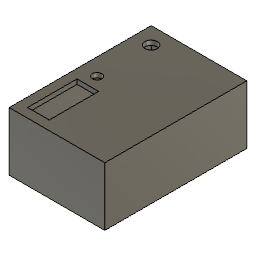
LocalMindCAD (Autodesk Fusion 360 design; units mm, degrees)
part number: 2026-03-10-18-57-42-287
Autodesk Fusion 360 part; units mm, degrees
sketch "Sketch1" plane through (0, 0, 0) normal (0, 0, 1) x (1, 0, 0)
  line L0 (31, 46) -> (-31, 46)
  line L1 (-31, 46) -> (-31, -46)
  line L2 (-31, -46) -> (31, -46)
  line L3 (31, -46) -> (31, 46)
  line L4 (31, 46) -> (-31, -46) construction
  line L5 (-31, 46) -> (31, -46) construction
  dimension "d1" = 62
  dimension "d2" = 92
  constraint horizontal L0
  constraint perpendicular L0 L1
  constraint parallel L0 L2
  constraint parallel L1 L3
  constraint coincident L4 origin
  constraint coincident L5 origin
  measures "d1" distance of L1.end L2.end
  measures "d2" distance of L0.end L1.end
extrude "Extrude1" add sketch "Sketch1" along normal blind 35
sketch "Sketch2" plane through (0, 0, 35) normal (0, 0, 1) x (-1, 0, 0)
  line L0 (-31, 46) -> (-31, -46)
  line L1 (-31, -46) -> (31, -46)
  line L2 (31, -46) -> (31, 46)
  line L3 (31, 46) -> (-31, 46)
  line L4 (31, 46) -> (-31, 46)
  line L5 (-31, 46) -> (-31, -46)
  line L6 (-31, -46) -> (31, -46)
  line L7 (31, -46) -> (31, 46)
  line L8 (29, -44) -> (29, 44)
  line L9 (29, 44) -> (-29, 44)
  line L10 (-29, 44) -> (-29, -44)
  line L11 (-29, -44) -> (29, -44)
  dimension "d5" = -2
  constraint horizontal L4
  constraint vertical L5
  constraint horizontal L6
  constraint vertical L7
  constraint coincident L0.end L1.start
  constraint coincident L2.end L3.start
extrude "Extrude2" cut sketch "Sketch2" against normal blind 33 contours L8 L9 L10 L11
sketch "Sketch3" plane through (0, 0, 2) normal (0, 0, 1) x (-1, 0, 0)
  line L0 (-29, -44) -> (29, -44)
  line L1 (29, -44) -> (29, 44)
  line L2 (29, 44) -> (-29, 44)
  line L3 (-29, 44) -> (-29, -44)
  line L4 (31, 46, 33) -> (-31, 46, 33)
  line L5 (-31, 46, 33) -> (-31, -46, 33)
  line L6 (-31, -46, 33) -> (31, -46, 33)
  line L7 (31, -46, 33) -> (31, 46, 33)
extrude "Extrude3" add sketch "Sketch3" along normal blind 3 contours L4 L5 L6 L7 in plane through (0, 0, 35) normal (0, 0, 1)
sketch "Sketch4" plane through (0, 0, 38) normal (0, 0, 1) x (-1, 0, 0)
  line L0 (31, -46) -> (31, 46)
  line L1 (31, 46) -> (-31, 46)
  line L2 (-31, 46) -> (-31, -46)
  line L3 (-31, -46) -> (31, -46)
  line L4 (25, 40) -> (11, 40)
  line L5 (11, 40) -> (11, 8)
  line L6 (11, 8) -> (25, 8)
  line L7 (25, 8) -> (25, 40)
  dimension "d10" = 14
  dimension "d11" = 32
  constraint horizontal L4
  constraint vertical L5
  constraint horizontal L6
  constraint vertical L7
  measures "d10" distance of L4.start L4.end
  measures "d11" distance of L4.start L6.end
extrude "Extrude4" cut sketch "Sketch4" against normal blind 3 contours L4 L5 L6 L7
sketch "Sketch5" plane through (0, 0, 38) normal (0, 0, 1) x (-1, 0, 0)
  line L0 (11, 40) -> (25, 40)
  line L1 (25, 40) -> (25, 8)
  line L2 (25, 8) -> (11, 8)
  line L3 (11, 8) -> (11, 40)
  line L4 (31, -46) -> (31, 46)
  line L5 (31, 46) -> (-31, 46)
  line L6 (-31, 46) -> (-31, -46)
  line L7 (-31, -46) -> (31, -46)
  circle A0 centre (20, 0) radius 3
  dimension "d14" = 6
  measures "d14" diameter of A0
extrude "Extrude5" cut sketch "Sketch5" against normal blind 3 contours A0
sketch "Sketch6" plane through (0, 0, 38) normal (0, 0, 1) x (-1, 0, 0)
  circle A0 centre (20, 0) radius 3
  line L0 (11, 40) -> (25, 40)
  line L1 (25, 40) -> (25, 8)
  line L2 (25, 8) -> (11, 8)
  line L3 (11, 8) -> (11, 40)
  line L4 (31, -46) -> (31, 46)
  line L5 (31, 46) -> (-31, 46)
  line L6 (-31, 46) -> (-31, -46)
  line L7 (-31, -46) -> (31, -46)
  circle A1 centre (20, -35) radius 4
  dimension "d17" = 8
  measures "d17" diameter of A1
extrude "Extrude6" cut sketch "Sketch6" against normal blind 3 contours A1
sketch "Sketch7" plane through (0, 0, 2) normal (0, 0, 1) x (-1, 0, 0)
  line L0 (-29, -44) -> (29, -44)
  line L1 (29, -44) -> (29, 44)
  line L2 (29, 44) -> (-29, 44)
  line L3 (-29, 44) -> (-29, -44)
  line L4 (-29.75, -36.75) -> (29.75, -36.75)
  line L5 (29.75, -36.75) -> (29.75, 36.75)
  line L6 (29.75, 36.75) -> (-29.75, 36.75)
  line L7 (-29.75, 36.75) -> (-29.75, -36.75)
  line L8 (-29.75, -36.75) -> (29.75, 36.75) construction
  line L9 (29.75, -36.75) -> (-29.75, 36.75) construction
  dimension "d20" = 59.5
  dimension "d21" = 73.5
  constraint horizontal L4
  constraint perpendicular L4 L5
  constraint parallel L4 L6
  constraint parallel L5 L7
  constraint coincident L8 origin
  constraint coincident L9 origin
  measures "d20" distance of L5.end L6.end
  measures "d21" distance of L4.end L5.end
extrude "Extrude7" add sketch "Sketch7" along normal blind 1.6 contours L1 L3 L4 L6
